Cam Halter (Autodesk Fusion 360 design; units mm, degrees)
Autodesk Fusion 360 part; units mm, degrees
sketch "Sketch1" plane through (0, 0, 0) normal (0, 0, 1) x (1, 0, 0)
  line L0 (0, 0) -> (74, 0)
  line L1 (74, 0) -> (74, 40)
  line L2 (74, 40) -> (0, 40)
  line L3 (0, 40) -> (0, 0)
  line L4 (0, 0) -> (74, 0)
  line L5 (74, 0) -> (74, 15)
  line L6 (74, 15) -> (0, 15)
  line L7 (0, 15) -> (0, 0)
  line L8 (0, 15) -> (8, 15)
  line L9 (8, 15) -> (8, 0)
  line L10 (8, 0) -> (0, 0)
  line L11 (0, 0) -> (0, 15)
  line L12 (74, 15) -> (66, 15)
  line L13 (66, 15) -> (66, 0)
  line L14 (66, 0) -> (74, 0)
  line L15 (74, 0) -> (74, 15)
  line L16 (8, 15) -> (66, 15)
  line L17 (66, 15) -> (66, 40)
  line L18 (66, 40) -> (8, 40)
  line L19 (8, 40) -> (8, 15)
  circle A0 centre (4, 30) radius 1.3
  circle A1 centre (70, 30) radius 1.3
  circle A2 centre (37, 7.5) radius 1.3
  dimension "d1" = 74
  dimension "d2" = 40
  dimension "d3" = 15
  dimension "d6" = 8
  dimension "d7" = 8
  dimension "d16" = 2.6
  dimension "d17" = 4
  dimension "d18" = 2.6
  dimension "d19" = 4
  dimension "d20" = 10
  dimension "d21" = 10
  dimension "d22" = 2.6
  dimension "d23" = 7.5
  dimension "d24" = 37
  dimension "d35" = 8
  constraint horizontal L0
  constraint vertical L1
  constraint horizontal L2
  constraint vertical L3
  constraint coincident L0.start L3.end
  constraint horizontal L4
  constraint vertical L5
  constraint horizontal L6
  constraint vertical L7
  constraint coincident L1 L5.end
  constraint horizontal L8
  constraint vertical L9
  constraint horizontal L10
  constraint vertical L11
  constraint horizontal L12
  constraint vertical L13
  constraint horizontal L14
  constraint vertical L15
  constraint horizontal L16
  constraint vertical L17
  constraint horizontal L18
  constraint vertical L19
  constraint coincident L2 L17.end
  measures "d1" distance of L0.start L0.end
  measures "d2" distance of L0.start L2.end
  measures "d3" distance of L0.start L6.end
  measures "d6" distance of L6.end L8.end
  measures "d7" distance of L5.end L12.end
  measures "d16" diameter of A0
  measures "d17" distance of L3 A0.centre
  measures "d18" diameter of A1
  measures "d19" distance of L1 A1.centre
  measures "d20" distance of L2 A1.centre
  measures "d21" distance of L2 A0.centre
  measures "d22" diameter of A2
  measures "d23" distance of L0 A2.centre
  measures "d24" distance of L3 A2.centre
  measures "d35" distance of L1 L17
extrude "Extrude1" add sketch "Sketch1" along normal blind 2 contours L0 L3 L4 L6 L7 L8 L9 L10 L11 | L0 L4 L6 L9 L13 L16 | L2 L3 L6 L8 L19 | L0 L1 L4 L5 L6 L12 L13 L14 L15 | L2 L6 L16 L17 L18 L19 | L1 L2 L6 L12 L17 | A0 | A1 | A2
extrude "Extrude5" add sketch "Sketch1" along normal blind 12 contours L2 L6 L16 L17 L18 L19
chamfer "Chamfer1" distance 20 distance2 10 1 edges at (37, 15, 12) measured on face at (27.3333, 31.6667, 12)
extrude "Extrude2" add sketch "Sketch1" along normal blind 25 contours L0 L3 L4 L6 L7 L8 L9 L10 L11 | L0 L1 L4 L5 L6 L12 L13 L14 L15
sketch "Sketch2" plane through (74, 0, 0) normal (1, 0, 0) x (0, 1, 0)
  line L0 (0, 0) -> (40, 0)
  line L1 (40, 0) -> (40, 2)
  line L2 (40, 2) -> (15, 2)
  line L3 (15, 2) -> (15, 25)
  line L4 (15, 25) -> (0, 25)
  line L5 (0, 25) -> (0, 0)
  line L6 (2.5, 22.5) -> (12.5, 22.5)
  line L7 (12.5, 22.5) -> (12.5, 15.5)
  line L8 (12.5, 15.5) -> (2.5, 15.5)
  line L9 (2.5, 15.5) -> (2.5, 22.5)
  dimension "d10" = 2.5
  dimension "d11" = 2.5
  dimension "d12" = 2.5
  dimension "d13" = 7
  constraint horizontal L6
  constraint vertical L7
  constraint horizontal L8
  constraint vertical L9
  measures "d10" distance of L4 L6
  measures "d11" distance of L5 L9
  measures "d12" distance of L3 L7
  measures "d13" distance of L6.start L8.end
extrude "Extrude3" cut sketch "Sketch2" against normal blind 100 contours L6 L7 L8 L9
extrude "Extrude4" cut sketch "Sketch1" along normal blind 10 contours A0 | A1 | A2
fillet "Fillet1" radius 3 4 edges at (70, 12.5, 22.5) (4, 12.5, 22.5) (70, 2.5, 22.5) (4, 2.5, 22.5)
fillet "Fillet2" radius 4 4 edges at (4, 15, 25) (4, 0, 25) (70, 0, 25) (70, 15, 25)
